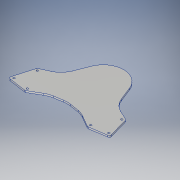
# Autodesk Inventor part: Ball Stop
Saved by Autodesk Inventor 2019.4 (Build 234330000, 330)
## iProperties
Created: 2020-01-06
Part Number: Ball Stop
Material: Aluminum 6061
Document SubType Name: Modeling
Designer: admin
Density: 2.7 g/cm^3
Appearance: Aluminum - Flat
Author: admin
Autodesk Inventor part; units mm, degrees
ref_plane "YZ Plane" through (0, 0, 0) normal (1, 0, 0) x (0, 1, 0)
ref_plane "XZ Plane" through (0, 0, 0) normal (0, 1, 0) x (-1, 0, 0)
ref_plane "XY Plane" through (0, 0, 0) normal (0, 0, 1) x (1, 0, 0)
sketch "Sketch1" plane through (0, 0, 0) normal (0, 1, 0) x (-1, 0, 0)
  line L0 (0, 0) -> (47.4827, 32.9139)
  line L1 (47.4827, 32.9139) -> (80.7316, 117.2675)
  line L2 (80.7316, 117.2675) -> (131.2206, 140.6648)
  line L3 (131.2206, 140.6648) -> (150, 206.2389)
  line L4 (150, 206.2389) -> (92.1224, 214.859)
  line L5 (92.1224, 214.859) -> (47.4827, 189.015)
  line L6 (47.4827, 189.015) -> (0, 180.9944)
  line L7 (0, 180.9944) -> (0, 0) construction
  line L8 (0, 0) -> (-47.4827, 32.9139)
  line L9 (-47.4827, 32.9139) -> (-80.7316, 117.2675)
  line L10 (-80.7316, 117.2675) -> (-131.2206, 140.6648)
  line L11 (-131.2206, 140.6648) -> (-150, 206.2389)
  line L12 (-150, 206.2389) -> (-92.1224, 214.859)
  line L13 (-92.1224, 214.859) -> (-47.4827, 189.015)
  line L14 (-47.4827, 189.015) -> (0, 180.9944)
  dimension "d0" = 150
  constraints: 30 end point, 6 symmetric about line, 1 vertical
  measures "d0" distance from line of L7 L3.end
extrude "Extrusion1" add sketch "Sketch1" along normal blind 5
sketch "Sketch2" plane through (0, 5, 0) normal (0, 1, 0) x (1, 0, 0)
  line L0 (0, 0) -> (-47.4827, -32.9139) projected
  line L1 (-47.4827, -32.9139) -> (-80.7316, -117.2675) projected
  line L2 (-80.7316, -117.2675) -> (-131.2206, -140.6648) projected
  line L3 (-131.2206, -140.6648) -> (-150, -206.2389) projected
  line L4 (-150, -206.2389) -> (-92.1224, -214.859) projected
  line L5 (-92.1224, -214.859) -> (-47.4827, -189.015) projected
  line L6 (-47.4827, -189.015) -> (0, -180.9944) projected
  line L7 (0, -180.9944) -> (47.4827, -189.015) projected
  line L8 (47.4827, -189.015) -> (92.1224, -214.859) projected
  line L9 (92.1224, -214.859) -> (150, -206.2389) projected
  line L10 (150, -206.2389) -> (131.2206, -140.6648) projected
  line L11 (131.2206, -140.6648) -> (80.7316, -117.2675) projected
  line L12 (80.7316, -117.2675) -> (47.4827, -32.9139) projected
  line L13 (47.4827, -32.9139) -> (0, 0) projected
  line L14 (-142.7598, -199.1184) -> (-127.3897, -145.449) construction
  line L15 (-125.9022, -143.711) -> (-76.8137, -120.9627)
  line L16 (-76.8137, -120.9627) -> (-43.3874, -36.1589)
  line L17 (-43.3874, -36.1589) -> (0, -6.0838)
  line L18 (0, -6.0838) -> (43.3874, -36.1589)
  line L19 (43.3874, -36.1589) -> (76.8137, -120.9627)
  line L20 (76.8137, -120.9627) -> (127.0434, -144.2398)
  line L21 (127.0434, -144.2398) -> (143.6233, -202.1335)
  line L22 (143.6233, -202.1335) -> (93.1148, -209.656)
  line L23 (93.1148, -209.656) -> (49.2062, -184.2353)
  line L24 (49.2062, -184.2353) -> (0, -175.9236)
  line L25 (0, -175.9236) -> (-49.2062, -184.2353)
  line L26 (-49.2062, -184.2353) -> (-92.2827, -209.1743)
  line L27 (-94.0657, -209.5144) -> (-140.5212, -202.5955) construction
  arc A0 (-142.7598, -199.1184) -> (-140.5212, -202.5955) centre (-140.1161, -199.8755) ccw
  arc A1 (-94.0657, -209.5144) -> (-92.2827, -209.1743) centre (-93.6606, -206.7944) ccw
  arc A2 (-125.9022, -143.711) -> (-127.3897, -145.449) centre (-124.746, -146.2061) ccw
  circle A3 centre (-93.6606, -206.7944) radius 2.75
  circle A4 centre (-140.1161, -199.8755) radius 2.75
  circle A5 centre (-124.746, -146.2061) radius 2.75
  dimension "d3" = 5
  dimension "d4" = 2.75
  dimension "d5" = 2.75
  dimension "d6" = 5.5
  dimension "d7" = 5.5
  dimension "d8" = 5.5
  constraints: 28 end point, 6 centre point, 6 point on circle, 6 tangent, 3 coincident, 1 equal radius, 13 other
  measures "d3" distance between parallel lines of L3 L14
  measures "d4" radius of A0
  measures "d5" radius of A2
  measures "d6" diameter of A3
  measures "d7" diameter of A4
  measures "d8" diameter of A5
extrude "Extrusion2" cut sketch "Sketch2" against normal through all contours A4 A0 | A3 A1 | A5 A2
mirror "Mirror1" about plane through (0, 0, 0) normal (1, 0, 0) of "Extrusion2"
fillet "Fillet1" radius 5 6 edges at (92.1224, 2.5, 214.859) (150, 2.5, 206.2389) (131.2206, 2.5, 140.6648) (-92.1224, 2.5, 214.859) (-150, 2.5, 206.2389) (-131.2206, 2.5, 140.6648)
fillet "Fillet2" radius 60 3 edges at (-47.4827, 2.5, 189.015) (0, 2.5, 180.9944) (47.4827, 2.5, 189.015)
fillet "Fillet3" radius 60 3 edges at (47.4827, 2.5, 32.9139) (0, 2.5, 0) (-47.4827, 2.5, 32.9139)
fillet "Fillet4" radius 60 2 edges at (80.7316, 2.5, 117.2675) (-80.7316, 2.5, 117.2675)
body "Solid1"
